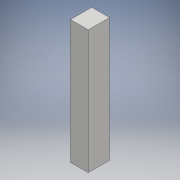
# Autodesk Inventor part: Dribbler block
Saved by Autodesk Inventor 2017 (Build 210142000, 142)
## iProperties
Created: 2017-03-27
Part Number: Dribbler block
Material: Generic
Document SubType Name: Modeling
Designer: yella
Density: 1 g/cm^3
Appearance: Default
Author: yella
Autodesk Inventor part; units mm, degrees
ref_plane "YZ Plane" through (0, 0, 0) normal (1, 0, 0) x (0, 1, 0)
ref_plane "XZ Plane" through (0, 0, 0) normal (0, 1, 0) x (-1, 0, 0)
ref_plane "XY Plane" through (0, 0, 0) normal (0, 0, 1) x (1, 0, 0)
sketch "Sketch1" plane through (0, 0, 0) normal (0, 1, 0) x (-1, 0, 0)
  line L0 (-5, 35) -> (-5, -35)
  line L1 (-5, -35) -> (5, -35)
  line L2 (5, -35) -> (5, 35)
  line L3 (5, 35) -> (-5, 35)
  line L4 (-5, 35) -> (5, -35) construction
  line L5 (-5, -35) -> (5, 35) construction
  point P0 (0, 0)
  dimension "d0" = 70
  dimension "d1" = 10
  constraints: 12 end point, 2 midpoint, 2 parallel, 1 perpendicular, 1 vertical
  measures "d0" distance of L0.start L0.end
  measures "d1" distance of L1.end L0.end
extrude "Extrusion1" add sketch "Sketch1" along normal blind 12
body "Solid1"
